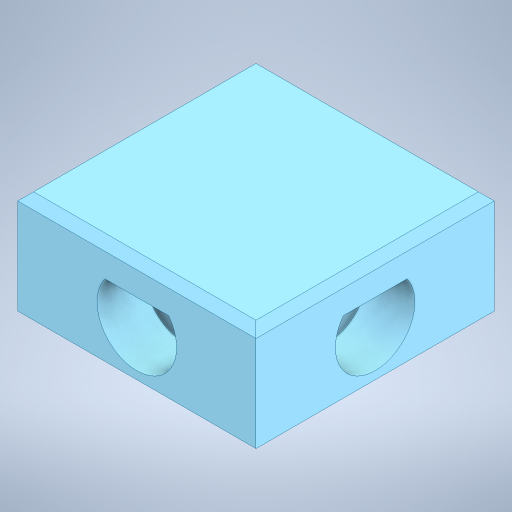
# Autodesk Inventor part: 몸통
Saved by Autodesk Inventor 2023 (Build 270158000, 158)
## iProperties
Created: 2022-10-29
Part Number: 몸통
Material: 일반
Document SubType Name: Modeling
Designer: 전상현
Density: 1 g/cm^3
Appearance: 기본값(1)
Author: 전상현
Autodesk Inventor part; units mm, degrees
ref_plane "YZ Plane" through (0, 0, 0) normal (1, 0, 0) x (0, 1, 0)
ref_plane "XZ Plane" through (0, 0, 0) normal (0, 1, 0) x (-1, 0, 0)
ref_plane "XY Plane" through (0, 0, 0) normal (0, 0, 1) x (1, 0, 0)
sketch "스케치1" plane through (0, 0, 0) normal (0, 1, 0) x (-1, 0, 0)
  line L0 (7.5, 7.5) -> (-7.5, 7.5)
  line L1 (-7.5, 7.5) -> (-7.5, -7.5)
  line L2 (-7.5, -7.5) -> (7.5, -7.5)
  line L3 (7.5, -7.5) -> (7.5, 7.5)
  line L4 (7.5, 7.5) -> (-7.5, -7.5) construction
  line L5 (-7.5, 7.5) -> (7.5, -7.5) construction
  point P0 (0, 0)
  dimension "d0" = 15
  dimension "d1" = 15
  constraints: 12 end point, 2 midpoint, 2 parallel, 1 horizontal, 1 perpendicular
  measures "d0" distance of L2.end L1.end
  measures "d1" distance of L0.end L1.end
extrude "돌출1" add sketch "스케치1" along normal blind 7
sketch "스케치2" plane through (-7.5, 0, 7.5) normal (0, 0, 1) x (1, 0, 0)
  circle A0 centre (7.5, 3.5) radius 2.5
  line L0 (0, 0) -> (15, 0) projected
  line L1 (0, 0) -> (0, 7) projected
  line L2 (5.5, 5) -> (9.5, 5)
  point P0 (7.5, 0)
  point P1 (7.5, 0)
  point P2 (0, 3.5)
  dimension "d5" = 5
  dimension "d14" = 1.5
  constraints: 2 end point, 2 midpoint, 2 point on circle, 1 centre point, 1 horizontal, 1 horizontal alignment, 1 vertical alignment
  measures "d5" diameter of A0
  measures "d14" distance from line of L2 A0.centre
chamfer "모따기1" distance 0.5 angle 45 8 edges at (0, 7, 7.5) (0, 0, 7.5) (7.5, 0, 0) (0, 0, -7.5) (-7.5, 0, 0) (-7.5, 7, 0) (0, 7, -7.5) (7.5, 7, 0)
extrude "돌출2" cut sketch "스케치2" against normal blind 3 contours A0 L2 picked at (8.1934, 3.1923)
pattern_circular "원형 패턴1" count 4 over 360 about axis through (0, -10, 0) along (0, 1, 0) of "돌출2"
